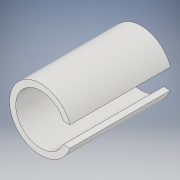
# Autodesk Inventor part: coupler
Saved by Autodesk Inventor 2017 (Build 210142000, 142)
## iProperties
Created: 2018-11-30
Part Number: coupler
Material: UHMW, White
Document SubType Name: Modeling
Designer: ddeboer
Density: 0.94 g/cm^3
Appearance: Smooth - White
Author: ddeboer
Autodesk Inventor part; units mm, degrees
ref_plane "YZ Plane" through (0, 0, 0) normal (1, 0, 0) x (0, 1, 0)
ref_plane "XZ Plane" through (0, 0, 0) normal (0, 1, 0) x (-1, 0, 0)
ref_plane "XY Plane" through (0, 0, 0) normal (0, 0, 1) x (1, 0, 0)
sketch "Sketch1" plane through (0, 0, 0) normal (0, 0, 1) x (1, 0, 0)
  circle A0 centre (0, 0) radius 16.713
  circle A1 centre (0, 0) radius 13.4
  dimension "d0" = 33.426
  dimension "d1" = 26.8
  constraints: 2 centre point, 2 coincident
  measures "d0" diameter of A0
  measures "d1" diameter of A1
extrude "Extrusion1" add sketch "Sketch1" along normal blind 53.9
sketch "Sketch2" plane through (0, 0, 53.9) normal (0, 0, 1) x (1, 0, 0)
  line L0 (15.7489, -5.5776) -> (19.7897, -5.5776)
  line L1 (19.7897, -5.5776) -> (19.7897, 5.4224)
  line L2 (19.7897, 5.4224) -> (15.7489, 5.4224)
  line L3 (15.7489, 5.4224) -> (15.7489, -5.5776)
  point P0 (0, 0)
  dimension "d4" = 11
  constraints: 8 end point, 2 parallel, 1 horizontal, 1 perpendicular
  measures "d4" distance of L0.end L1.end
extrude "Extrusion2" cut sketch "Sketch2" against normal blind 100
sketch "Sketch3" plane through (15.7489, -5.5776, 53.9) normal (1, 0, 0) x (0, 0, -1)
  line L0 (53.9, 0) -> (0, 0) projected
  line L1 (0, 11) -> (53.9, 11) projected
  line L2 (0, 0) -> (53.9, 0)
  line L3 (53.9, 0) -> (53.9, 11)
  line L4 (53.9, 11) -> (0, 11)
  line L5 (0, 11) -> (0, 0)
  point P0 (53.9, 5.5776)
  constraints: 8 end point, 2 parallel, 1 horizontal, 1 perpendicular
extrude "Extrusion3" cut sketch "Sketch3" against normal blind 10
body "Solid1"
